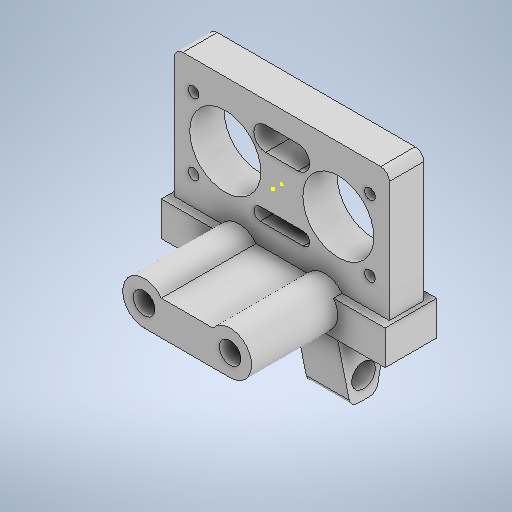
# Autodesk Inventor part: Czujnik_podstawa
Saved by Autodesk Inventor 2025.2 (Build 292293000, 293)
## iProperties
Created: 2025-11-25
Part Number: Czujnik_podstawa
Material: Ogólny
Document SubType Name: Modeling
Designer: juras
Density: 1 g/cm^3
Appearance: Domyślna
Author: juras
Autodesk Inventor part; units mm, degrees
ref_plane "YZ Plane" through (0, 0, 0) normal (1, 0, 0) x (0, 1, 0)
ref_plane "XZ Plane" through (0, 0, 0) normal (0, 1, 0) x (-1, 0, 0)
ref_plane "XY Plane" through (0, 0, 0) normal (0, 0, 1) x (1, 0, 0)
sketch "Szkic1" plane through (0, 0, 0) normal (0, 0, 1) x (1, 0, 0)
  line L0 (-25, -15) -> (25, -15)
  line L1 (25, -15) -> (25, 15)
  line L2 (25, 15) -> (-25, 15)
  line L3 (-25, 15) -> (-25, -15)
  line L4 (-25, -15) -> (25, 15) construction
  line L5 (25, -15) -> (-25, 15) construction
  point P0 (0, 0)
  dimension "d0" = 50
  dimension "d1" = 30
  constraints: 12 end point, 2 midpoint, 2 parallel, 1 horizontal, 1 perpendicular
  measures "d0" distance of L2.end L1.end
  measures "d1" distance of L1.end L0.end
extrude "Wyciągnięcie proste1" add sketch "Szkic1" along normal mid plane 8
sketch "Szkic8" plane through (0, 0, -4) normal (0, 0, -1) x (-1, 0, 0)
  line L0 (-20.5, -8.25) -> (20.5, -8.25)
  line L1 (20.5, -8.25) -> (20.5, 8.25)
  line L2 (20.5, 8.25) -> (-20.5, 8.25)
  line L3 (-20.5, 8.25) -> (-20.5, -8.25)
  line L4 (-20.5, -8.25) -> (20.5, 8.25) construction
  line L5 (20.5, -8.25) -> (-20.5, 8.25) construction
  point P0 (0, 0)
  dimension "d24" = 41
  dimension "d25" = 16.5
  constraints: 12 end point, 2 midpoint, 2 parallel, 1 horizontal, 1 perpendicular
  measures "d24" distance of L2.end L1.end
  measures "d25" distance of L0.end L1.end
hole "Otwór2" at (20.5, 8.25, -4) at (20.5, -8.25, -4) at (-20.5, 8.25, -4) at (-20.5, -8.25, -4) direction (0, 0, 1) diameter 2.5 depth 25 tip angle 118
sketch "Szkic9" plane through (0, 0, -4) normal (0, 0, -1) x (-1, 0, 0)
  line L0 (-22.5, -10) -> (22.5, -10)
  line L1 (22.5, -10) -> (22.5, 10)
  line L2 (22.5, 10) -> (-22.5, 10)
  line L3 (-22.5, 10) -> (-22.5, -10)
  line L4 (-22.5, -10) -> (22.5, 10) construction
  line L5 (22.5, -10) -> (-22.5, 10) construction
  circle A0 centre (-13.15, 0) radius 8.25
  line L6 (25, 15) -> (-25, 15) projected
  point P0 (0, 0)
  dimension "d33" = 45
  dimension "d34" = 20
  dimension "d35" = 16.5
  dimension "d36" = 9.35
  dimension "d38" = 10
  constraints: 12 end point, 2 midpoint, 2 parallel, 1 centre point, 1 horizontal, 1 perpendicular
  measures "d33" distance of L2.end L1.end
  measures "d34" distance of L1.end L0.end
  measures "d35" diameter of A0
  measures "d36" distance from line of A0.centre L3
  measures "d38" distance from line of A0.centre L2
extrude "Wyciągnięcie proste3" cut sketch "Szkic9" against normal blind 8 contours A0
mirror "Odbij1" about plane through (0, 0, 0) normal (1, 0, 0) of "Wyciągnięcie proste3"
sketch "Szkic10" plane through (0, 0, -4) normal (0, 0, -1) x (-1, 0, 0)
  line L0 (-22.5, -10) -> (22.5, -10)
  line L1 (22.5, -10) -> (22.5, 10)
  line L2 (22.5, 10) -> (-22.5, 10)
  line L3 (-22.5, 10) -> (-22.5, -10)
  line L4 (-22.5, -10) -> (22.5, 10) construction
  line L5 (22.5, -10) -> (-22.5, 10) construction
  line L6 (-3.75, 7.25) -> (3.75, 7.25) construction
  line L7 (-3.75, 10) -> (3.75, 10)
  line L8 (3.75, 4.5) -> (-3.75, 4.5)
  arc A0 (-3.75, 10) -> (-3.75, 4.5) centre (-3.75, 7.25) ccw
  arc A1 (3.75, 4.5) -> (3.75, 10) centre (3.75, 7.25) ccw
  line L9 (25, -15) -> (25, 15) projected
  line L10 (-5, -8.5) -> (5, -8.5) construction
  line L11 (-5, -10) -> (5, -10)
  line L12 (5, -7) -> (-5, -7)
  arc A2 (-5, -7) -> (-5, -10) centre (-5, -8.5) ccw
  arc A3 (5, -10) -> (5, -7) centre (5, -8.5) ccw
  point P0 (0, 0)
  point P1 (0, 7.25)
  point P2 (-6.5, 7.25)
  point P3 (6.5, 7.25)
  point P4 (0, -8.5)
  point P5 (-6.5, -8.5)
  point P6 (6.5, -8.5)
  point P7 (5, -10)
  point P8 (3.75, 10)
  dimension "d41" = 45
  dimension "d42" = 20
  dimension "d43" = 0
  dimension "d44" = 5.5
  dimension "d45" = 16
  dimension "d47" = 16
  dimension "d48" = 0
  dimension "d49" = 3
  dimension "d50" = 16
  dimension "d51" = 16
  constraints: 28 end point, 12 point on circle, 8 tangent, 4 centre point, 4 midpoint, 4 parallel, 3 horizontal, 1 perpendicular
  measures "d41" distance of L2.end L1.end
  measures "d42" distance of L1.end L0.end
  measures "d43" distance between parallel lines of L2 L7
  measures "d44" distance between parallel lines of L2 L8
  measures "d45" distance from line of L3 point (-6.5, 7.25)
  measures "d47" distance from line of L1 point (6.5, 7.25)
  measures "d48" distance between parallel lines of L0 L11
  measures "d49" distance between parallel lines of L0 L12
  measures "d50" distance from line of L3 point (-6.5, -8.5)
  measures "d51" distance from line of L1 point (6.5, -8.5)
extrude "Wyciągnięcie proste4" cut sketch "Szkic10" against normal blind 8 contours A2 L12 A3 L0 | L2 A1 L8 A0
fillet "Zaokrąglenie1" radius 2 2 edges at (25, 15, 0) (-25, 15, 0)
sketch "Szkic11" plane through (-25, -15, 4) normal (0, -1, 0) x (1, 0, 0)
  line L0 (51, -10) -> (-1, -10)
  line L1 (-1, -10) -> (-1, 2)
  line L2 (-1, 2) -> (51, 2)
  line L3 (51, 2) -> (51, -10)
  line L4 (51, -10) -> (-1, 2) construction
  line L5 (-1, -10) -> (51, 2) construction
  line L6 (50, -8) -> (0, -8) projected
  line L7 (0, -8) -> (0, 0) projected
  point P0 (25, -4)
  dimension "d55" = 2
  dimension "d57" = 52
  constraints: 12 end point, 2 midpoint, 2 parallel, 1 horizontal, 1 perpendicular
  measures "d55" distance between parallel lines of L6 L0
  measures "d57" distance of L1.end L2.end
extrude "Wyciągnięcie proste5" add sketch "Szkic11" along normal blind 8
sketch "Szkic13" plane through (-25, -23, 4) normal (0, -1, 0) x (1, 0, 0)
  line L0 (40, 2) -> (30, 2)
  line L1 (30, 2) -> (30, -10)
  line L2 (30, -10) -> (40, -10)
  line L3 (40, -10) -> (40, 2)
  line L4 (40, 2) -> (30, -10) construction
  line L5 (30, 2) -> (40, -10) construction
  line L6 (-1, -10) -> (51, -10) projected
  line L7 (51, 2) -> (-1, 2) projected
  point P0 (25, -4)
  point P1 (35, -4)
  dimension "d63" = 5
  dimension "d64" = 10
  dimension "d65" = 0
  dimension "d66" = 0
  constraints: 12 end point, 2 midpoint, 2 parallel, 1 horizontal, 1 perpendicular
  measures "d63" distance from line of point (25, -4) L1
  measures "d64" distance of L1.end L2.end
  measures "d65" distance between parallel lines of L6 L2
  measures "d66" distance between parallel lines of L7 L0
extrude "Wyciągnięcie proste6" add sketch "Szkic13" along normal blind 15
sketch "Szkic14" plane through (5, -23, -6) normal (-1, 0, 0) x (0, 0, 1)
  circle A0 centre (6, -10) radius 2.75
  line L0 (12, -15) -> (0, -15) projected
  line L1 (0, 0) -> (0, -15) projected
  point P0 (6, 23)
  dimension "d69" = 5.5
  dimension "d70" = 5
  dimension "d71" = 6
  constraints: 1 centre point
  measures "d69" diameter of A0
  measures "d70" distance from line of A0.centre L0
  measures "d71" distance from line of L1 A0.centre
extrude "Wyciągnięcie proste7" cut sketch "Szkic14" against normal blind 15
sketch "Szkic15" plane through (5, -23, -6) normal (-1, 0, 0) x (0, 0, 1)
  line L0 (0, 0) -> (12, 0) projected
  line L1 (0, 0) -> (0, -15) projected
  line L2 (0, 0) -> (0, -15)
  line L3 (12, -15) -> (0, -15) projected
  line L4 (0, -15) -> (3, -15)
  line L5 (3, -15) -> (0, 0)
  point P0 (6, 23)
  dimension "d74" = 3
  constraints: 6 end point, 1 collinear, 1 point on line
  measures "d74" distance of L1.end L4.end
extrude "Wyciągnięcie proste8" cut sketch "Szkic15" against normal blind 15
sketch "Szkic16" plane through (5, -38, 6) normal (-1, 0, 0) x (0, 0, 1)
  line L0 (-12, 15) -> (0, 15) projected
  line L1 (0, 15) -> (0, 0) projected
  line L2 (0, 15) -> (0, 0)
  line L3 (0, 0) -> (-3, 0)
  line L4 (-3, 0) -> (0, 15)
  point P0 (-6, 38)
  dimension "d77" = 3
  constraints: 6 end point, 1 collinear, 1 perpendicular
  measures "d77" distance of L1.end L3.end
extrude "Wyciągnięcie proste9" cut sketch "Szkic16" against normal blind 15
fillet "Zaokrąglenie2" radius 2 2 edges at (10, -38, -3) (10, -38, 3)
mirror "Odbij2" about plane through (0, 0, 0) normal (1, 0, 0) of "Wyciągnięcie proste6", "Wyciągnięcie proste7", "Wyciągnięcie proste8", "Wyciągnięcie proste9", "Zaokrąglenie2"
sketch "Szkic22" plane through (-26, -15, 6) normal (0, 0, 1) x (1, 0, 0)
  line L0 (8, -8) -> (44, -8)
  line L1 (44, -8) -> (44, 0)
  line L2 (44, 0) -> (8, 0)
  line L3 (8, 0) -> (8, -8)
  line L4 (8, -8) -> (44, 0) construction
  line L5 (44, -8) -> (8, 0) construction
  line L6 (0, 0) -> (0, -8) projected
  line L7 (52, 0) -> (52, -8) projected
  line L8 (52, 0) -> (0, 0) projected
  circle A0 centre (16, -3) radius 5
  circle A1 centre (16, -3) radius 2.5
  circle A2 centre (36, -3) radius 5
  line L9 (41, -8) -> (31, -8) projected
  circle A3 centre (36, -3) radius 2.5
  point P0 (26, 15)
  point P1 (26, -4)
  point P2 (20, 0)
  point P3 (16, -8)
  point P4 (36, -8)
  point P5 (32, 0)
  dimension "d109" = 8
  dimension "d110" = 8
  dimension "d111" = 8
  dimension "d112" = 0
  dimension "d113" = 5
  dimension "d114" = 10
  dimension "d115" = 8
  dimension "d116" = 5
  dimension "d123" = 8
  dimension "d124" = 10
  dimension "d125" = 5
  constraints: 12 end point, 4 centre point, 2 coincident, 2 midpoint, 2 parallel, 1 horizontal, 1 perpendicular, 1 tangent
  measures "d109" distance between parallel lines of L6 L3
  measures "d110" distance between parallel lines of L7 L1
  measures "d111" distance between parallel lines of L0 L2
  measures "d112" distance between parallel lines of L8 L2
  measures "d113" distance from line of L0 A0.centre
  measures "d114" diameter of A0
  measures "d115" distance from line of A0.centre L3
  measures "d116" diameter of A1
  measures "d123" distance from line of L1 A2.centre
  measures "d124" diameter of A2
  measures "d125" diameter of A3
extrude "Wyciągnięcie proste13" add sketch "Szkic22" along normal blind 20 contours L0 A0 L2 A2 | A2 L2 | A2 L2 | A0 L2 | L2 A0
sketch "Szkic23" plane through (-26, -15, 6) normal (0, 0, -1) x (-1, 0, 0)
  point P0 (-26, 15)
sketch "Szkic24" plane through (0, 0, 4) normal (0, 0, 1) x (1, 0, 0)
  point P0 (0, 0)
sketch "Szkic25" plane through (0, 0, 4) normal (0, 0, 1) x (1, 0, 0)
  circle A0 centre (-10, -18) radius 2.5 projected
  circle A1 centre (-10, -18) radius 5
  point P0 (0, 0)
  dimension "d128" = 10
  constraints: 1 centre point, 1 coincident
  measures "d128" diameter of A1
extrude "Wyciągnięcie proste14" add sketch "Szkic25" along normal blind 2
mirror "Odbij4" about plane through (0, 0, 0) normal (1, 0, 0) of "Wyciągnięcie proste14"
